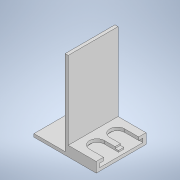
# Autodesk Inventor part: prototype7_1
Saved by Autodesk Inventor 2022 (Build 260153000, 153)
## iProperties
Created: 2022-06-15
Part Number: prototype7_1
Material: Generic
Document SubType Name: Modeling
Designer: tecware
Density: 1 g/cm^3
Appearance: Default
Author: tecware
Autodesk Inventor part; units mm, degrees
ref_plane "YZ Plane" through (0, 0, 0) normal (1, 0, 0) x (0, 1, 0)
ref_plane "XZ Plane" through (0, 0, 0) normal (0, 1, 0) x (-1, 0, 0)
ref_plane "XY Plane" through (0, 0, 0) normal (0, 0, 1) x (1, 0, 0)
sketch "Sketch1" plane through (0, 0, 0) normal (0, 1, 0) x (-1, 0, 0)
  line L0 (9, -16) -> (-9, -16)
  line L1 (-9, -16) -> (-9, 16)
  line L2 (-9, 16) -> (9, 16)
  line L3 (9, 16) -> (9, -16)
  line L4 (9, -16) -> (-9, 16) construction
  line L5 (-9, -16) -> (9, 16) construction
  circle A0 centre (0, 6.5) radius 4.8
  line L6 (0, 6.5) -> (0, -6.5)
  circle A1 centre (0, -6.5) radius 4.8
  line L7 (0, 11.3) -> (-9, 11.3)
  line L8 (0, 1.7) -> (-9, 1.7)
  line L9 (0, -1.7) -> (-9, -1.7)
  line L10 (0, -11.3) -> (-9, -11.3)
  point P0 (0, 0)
  point P1 (0, 0)
  dimension "d0" = 18
  dimension "d1" = 32
  dimension "d2" = 9.6
  dimension "d3" = 13
  dimension "d4" = 9.6
  constraints: 22 end point, 6 point on line, 4 point on circle, 3 midpoint, 2 centre point, 1 coincident
  measures "d0" distance of L1.end L2.end
  measures "d1" distance of L0.end L1.end
  measures "d2" diameter of A0
  measures "d3" distance of L6.start L6.end
  measures "d4" diameter of A1
extrude "Extrusion1" add sketch "Sketch1" along normal blind 2 contours L0 L1 L10 A1 L6 A0 L7 L2 L3 | L1 L8 L6 L9
sketch "Sketch2" plane through (0, 0, 0) normal (0, -1, 0) x (1, 0, 0)
  line L0 (-9, 16) -> (9, 16) projected
  line L1 (9, 16) -> (-9, 16)
  line L2 (-9, -16) -> (-9, 16) projected
  line L3 (-9, 16) -> (-9, -16)
  line L4 (9, -16) -> (-9, -16) projected
  line L5 (-9, -16) -> (9, -16)
  line L6 (9, -16) -> (9, -14)
  line L7 (9, -11.3) -> (9, -16) projected
  line L8 (9, -14) -> (-7, -14)
  line L9 (-7, -14) -> (-7, 14)
  line L10 (-7, 14) -> (9, 14)
  line L11 (9, 16) -> (9, 11.3) projected
  point P0 (0, 0)
  dimension "d7" = 2
  dimension "d8" = 16
  dimension "d9" = 28
  constraints: 14 end point, 2 point on line
  measures "d7" distance of L4.start L6.end
  measures "d8" distance of L6.end L8.end
  measures "d9" distance of L8.end L9.end
extrude "Extrusion2" add sketch "Sketch2" along normal blind 2.5
sketch "Sketch3" plane through (-9, 2, -16) normal (-1, 0, 0) x (0, 0, 1)
  line L0 (0, 0) -> (0, -4.5) projected
  line L1 (0, -4.5) -> (32, -4.5)
  line L2 (32, -4.5) -> (32, 50)
  line L3 (32, 50) -> (0, 50)
  line L4 (0, 50) -> (0, -4.5)
  point P0 (16, -2)
  dimension "d12" = 54.5
  constraints: 8 end point
  measures "d12" distance of L2.end L1.end
extrude "Extrusion3" add sketch "Sketch3" along normal blind 2
sketch "Sketch4" plane through (0, -2.5, 0) normal (0, -1, 0) x (1, 0, 0)
  line L0 (9, 16) -> (9, 11.3) projected
  line L1 (9, 16) -> (-31, 16)
  line L2 (-31, 16) -> (-31, -16)
  line L3 (-31, -16) -> (9, -16)
  line L4 (9, -16) -> (9, 16)
  point P0 (0, 0)
  dimension "d15" = 40
  constraints: 8 end point
  measures "d15" distance of L3.end L2.end
extrude "Extrusion4" add sketch "Sketch4" along normal blind 2
sketch "Sketch5" plane through (-7, 0, 14) normal (1, 0, 0) x (0, 0, -1)
  line L0 (0, 0) -> (0, -2.5) projected
  line L1 (30, -2.5) -> (-2, -2.5) projected
  line L2 (0, 0) -> (3, 0)
  line L3 (3, 0) -> (3, -2.5)
  line L4 (3, -2.5) -> (0, -2.5)
  line L5 (0, -2.5) -> (0, 0)
  point P0 (14, 0)
  dimension "d18" = 3
  constraints: 8 end point, 1 point on line
  measures "d18" distance of L3.end L4.end
extrude "Extrusion5" cut sketch "Sketch5" against normal up to surface (4 mm away)
sketch "Sketch6" plane through (9, 0, 1.7) normal (1, 0, 0) x (0, 0, -1)
  line L0 (0, 0) -> (0, 2) projected
  line L1 (3.4, 0) -> (3.4, 2) projected
  line L2 (0, 1) -> (3.4, 1)
  line L3 (3.4, 1) -> (3.4, 2)
  line L4 (3.4, 2) -> (0, 2)
  line L5 (0, 2) -> (0, 1)
  point P0 (1.7, 0)
  constraints: 8 end point, 1 midpoint
extrude "Extrusion6" cut sketch "Sketch6" against normal blind 2.2
body "Solid1"
